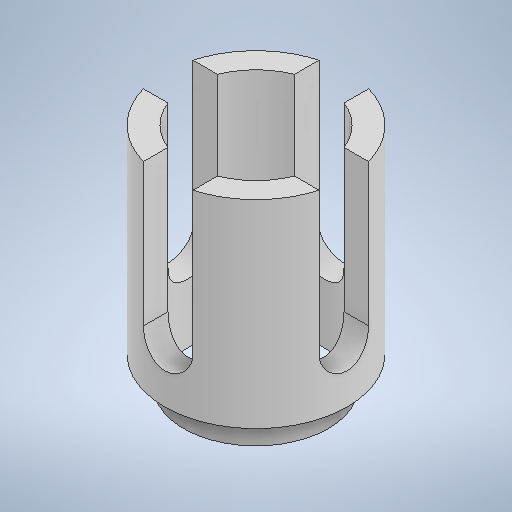
# Autodesk Inventor part: trava_botao
Saved by Autodesk Inventor 2025.3 (Build 293356000, 356)
## iProperties
Created: 2025-07-27
Part Number: trava_botao
Material: Genérico
Document SubType Name: Modeling
Designer: user
Density: 1 g/cm^3
Appearance: Padrão
Author: user
## iProperties of the stored document trava_botao_3DPrint.ipt
Created: 2025-07-28
Part Number: trava_botao_3DPrint
Material: Genérico
Document SubType Name: Modeling
Designer: user
Density: 1 g/cm^3
Appearance: Padrão
Author: user
Autodesk Inventor part; units mm, degrees
ref_plane "XZ Plane" through (0, 0, 0) normal (0, 1, 0) x (-1, 0, 0)
sketch "Esboço1" plane through (0, 0, 0) normal (0, 0, 1) x (1, 0, 0)
  line L0 (0, 0) -> (7.3, 0)
  line L1 (7.3, 0) -> (7.3, 2.85)
  line L2 (7.3, 2.85) -> (9.2, 2.85)
  line L3 (0, 22.85) -> (0, 0)
  line L4 (9.2, 2.85) -> (9.2, 6.85)
  line L5 (6.85, 0) -> (6.85, 22.85)
  line L6 (9.2, 6.85) -> (9.2, 22.85)
  line L7 (9.2, 6.85) -> (9.2, 6.85)
  line L8 (9.2, 22.85) -> (0, 22.85)
  dimension "d0" = 7.3
  dimension "d1" = 2.85
  dimension "d4" = 4
  dimension "d7" = 9.2
  dimension "d11" = 2.35
  dimension "d12" = 9.2
  dimension "d24" = 16
  constraints: 18 end point, 4 horizontal, 1 perpendicular, 1 point on line, 1 vertical
  measures "d0" distance of L0.start L0.end
  measures "d1" distance of L0.end L1.end
  measures "d4" distance of L2.end L4.end
  measures "d7" distance between parallel lines of L3 L4
  measures "d11" distance between parallel lines of L6 L5
  measures "d12" distance between parallel lines of L3 L6
  measures "d24" distance of L6.start L6.end
revolve "Revolução1" add sketch "Esboço1" angle 360 about axis through (0, 22.85, 0) along (0, -1, 0) contours L5 L8 L6 L4 L2 L1 L0
ref_plane "Plano de trabalho1" through (0, 12.85, 9.2) normal (0, 0, 1) x (1, 0, 0)
sketch "Esboço3" plane through (0, 12.85, 9.2) normal (0, 0, 1) x (1, 0, 0)
  line L0 (0, -12.85) -> (0, -6.85)
  line L1 (-9.2, 10) -> (9.2, 10) projected
  line L2 (0, -6.85) -> (0, -4.35)
  arc A0 (-2.5, -4.35) -> (2.5, -4.35) centre (0, -4.35) ccw
  line L3 (2.5, -4.35) -> (2.5, 10)
  line L4 (-2.5, -4.35) -> (-2.5, 10)
  point P0 (-2, 10)
  point P1 (2, 10)
  dimension "d16" = 6
  dimension "d25" = 2.5
  constraints: 8 end point, 4 point on line, 4 vertical, 3 point on circle, 2 tangent, 1 centre point, 1 coincident
  measures "d16" distance of L0.start L0.end
  measures "d25" distance of L0.end L2.end
ref_plane "Plano de trabalho2" through (-9.2, 12.85, 0) normal (1, 0, 0) x (0, 1, 0)
sketch "Esboço4" plane through (-9.2, 12.85, 0) normal (1, 0, 0) x (0, 1, 0)
  line L0 (-12.85, 0) -> (-6.85, 0)
  line L1 (10, 0) -> (10, 0) projected
  line L2 (10, -2) -> (10, 2)
  line L3 (10, 0) -> (10, 0) projected
  arc A0 (-4.35, 2.5) -> (-4.35, -2.5) centre (-4.35, 0) ccw
  line L4 (-4.35, 2.5) -> (10, 2.5)
  line L5 (-4.35, -2.5) -> (10, -2.5)
  line L6 (10, -2.5) -> (10, 2.5)
  dimension "d20" = 6
  constraints: 10 end point, 4 point on line, 3 horizontal, 3 point on circle, 2 tangent, 1 centre point, 1 collinear, 1 vertical
  measures "d20" distance of L0.start L0.end
extrude "Extrusão3" cut sketch "Esboço3" against normal blind 20
extrude "Extrusão4" cut sketch "Esboço4" along normal blind 20
